kontentkelder (Autodesk Fusion 360 design; units mm, degrees)
Autodesk Fusion 360 part; units mm, degrees
sketch "Sketch1" plane through (0, 0, 0) normal (0, 0, 1) x (1, 0, 0)
  line L0 (0, 0) -> (-148, 0)
  line L1 (-148, 0) -> (-148, 42)
  line L2 (-148, 42) -> (0, 42)
  line L3 (0, 42) -> (0, 0)
  line L4 (-133.4456, 20.7821) -> (-135.5599, 20.7821)
  line L5 (-135.5599, 20.7821) -> (-135.5599, 23.5325)
  line L6 (-135.5599, 23.5325) -> (-136.4022, 23.5325)
  line L7 (-136.4022, 23.5325) -> (-137.9063, 26.7899)
  spline S0 degree 2 poles (-137.9063, 26.7899) (-137.9407, 26.8587) (-138.0524, 27.0563) knots 0 0 0 1 1 1
  spline S1 degree 2 poles (-138.0524, 27.0563) (-138.1126, 27.1595) (-138.3704, 27.6494) knots 0 0 0 1 1 1
  spline S2 degree 2 poles (-138.3704, 27.6494) (-138.8001, 28.4573) (-139.0236, 28.6808) knots 0 0 0 1 1 1
  spline S3 degree 2 poles (-139.0236, 28.6808) (-139.4018, 29.0417) (-140.1323, 29.0503) knots 0 0 0 1 1 1
  line L8 (-140.1323, 29.0503) -> (-140.1323, 23.5325)
  line L9 (-140.1323, 23.5325) -> (-142.6764, 23.5325)
  line L10 (-142.6764, 23.5325) -> (-142.6764, 36.1325)
  line L11 (-142.6764, 36.1325) -> (-140.1323, 36.1325)
  line L12 (-140.1323, 36.1325) -> (-140.1323, 30.7693)
  spline S4 degree 2 poles (-140.1323, 30.7693) (-139.1783, 30.8638) (-138.7228, 31.5514) knots 0 0 0 1 1 1
  spline S5 degree 2 poles (-138.7228, 31.5514) (-138.6111, 31.7405) (-138.0524, 33.1673) knots 0 0 0 1 1 1
  spline S6 degree 2 poles (-138.0524, 33.1673) (-137.3304, 35.0323) (-136.6085, 35.591) knots 0 0 0 1 1 1
  spline S7 degree 2 poles (-136.6085, 35.591) (-135.8091, 36.2098) (-133.9097, 36.2098) knots 0 0 0 1 1 1
  spline S8 degree 2 poles (-133.9097, 36.2098) (-133.8237, 36.2098) (-133.5401, 36.2184) knots 0 0 0 1 1 1
  line L13 (-133.5401, 36.2184) -> (-133.5401, 34.3362)
  line L14 (-133.5401, 34.3362) -> (-133.9011, 34.3447)
  spline S9 degree 2 poles (-133.9011, 34.3447) (-135.1731, 34.3791) (-135.6286, 33.5626) knots 0 0 0 1 1 1
  spline S10 degree 2 poles (-135.6286, 33.5626) (-135.8521, 33.1673) (-136.2905, 31.9382) knots 0 0 0 1 1 1
  spline S11 degree 2 poles (-136.2905, 31.9382) (-136.5655, 31.1647) (-136.8147, 30.8209) knots 0 0 0 1 1 1
  spline S12 degree 2 poles (-136.8147, 30.8209) (-137.1241, 30.3739) (-137.7516, 30.0216) knots 0 0 0 1 1 1
  spline S13 degree 2 poles (-137.7516, 30.0216) (-136.8921, 29.7809) (-136.342, 29.0503) knots 0 0 0 1 1 1
  spline S14 degree 2 poles (-136.342, 29.0503) (-135.7232, 28.2338) (-135.1301, 26.9876) knots 0 0 0 1 1 1
  line L15 (-135.1301, 26.9876) -> (-134.4941, 25.6468)
  line L16 (-134.4941, 25.6468) -> (-133.4456, 25.6468)
  line L17 (-133.4456, 25.6468) -> (-133.4456, 20.7821)
  line L18 (-122.6075, 35.2128) -> (-121.2495, 36.7341)
  line L19 (-121.2495, 36.7341) -> (-120.0548, 35.6855)
  line L20 (-120.0548, 35.6855) -> (-121.4902, 34.0697)
  spline S15 degree 2 poles (-121.4902, 34.0697) (-120.9143, 33.2962) (-120.5963, 32.166) knots 0 0 0 1 1 1
  spline S16 degree 2 poles (-120.5963, 32.166) (-120.2783, 31.0357) (-120.2783, 29.7637) knots 0 0 0 1 1 1
  spline S17 degree 2 poles (-120.2783, 29.7637) (-120.2783, 26.7641) (-121.9371, 25.0409) knots 0 0 0 1 1 1
  spline S18 degree 2 poles (-121.9371, 25.0409) (-123.5959, 23.3176) (-126.3205, 23.3176) knots 0 0 0 1 1 1
  spline S19 degree 2 poles (-126.3205, 23.3176) (-128.684, 23.3176) (-130.1022, 24.392) knots 0 0 0 1 1 1
  line L21 (-130.1022, 24.392) -> (-131.4945, 22.8277)
  line L22 (-131.4945, 22.8277) -> (-132.715, 23.8935)
  line L23 (-132.715, 23.8935) -> (-131.2453, 25.5437)
  spline S20 degree 2 poles (-131.2453, 25.5437) (-132.5001, 27.2196) (-132.5001, 29.9098) knots 0 0 0 1 1 1
  spline S21 degree 2 poles (-132.5001, 29.9098) (-132.5001, 32.8922) (-130.8413, 34.6198) knots 0 0 0 1 1 1
  spline S22 degree 2 poles (-130.8413, 34.6198) (-129.1825, 36.3473) (-126.415, 36.3473) knots 0 0 0 1 1 1
  spline S23 degree 2 poles (-126.415, 36.3473) (-124.1202, 36.3473) (-122.6075, 35.2128) knots 0 0 0 1 1 1
  spline S24 degree 2 poles (-124.1889, 33.4423) (-125.057, 34.1814) (-126.3892, 34.1814) knots 0 0 0 1 1 1
  spline S25 degree 2 poles (-126.3892, 34.1814) (-127.9535, 34.1814) (-128.9161, 33.1028) knots 0 0 0 1 1 1
  spline S26 degree 2 poles (-128.9161, 33.1028) (-129.8787, 32.0241) (-129.8787, 29.8497) knots 0 0 0 1 1 1
  spline S27 degree 2 poles (-129.8787, 29.8497) (-129.8787, 28.4831) (-129.4834, 27.5119) knots 0 0 0 1 1 1
  line L24 (-129.4834, 27.5119) -> (-124.1889, 33.4423)
  line L25 (-123.2521, 32.0929) -> (-128.5379, 26.1539)
  spline S28 degree 2 poles (-128.5379, 26.1539) (-127.6527, 25.3804) (-126.4064, 25.3804) knots 0 0 0 1 1 1
  spline S29 degree 2 poles (-126.4064, 25.3804) (-124.8765, 25.3804) (-123.8924, 26.4891) knots 0 0 0 1 1 1
  spline S30 degree 2 poles (-123.8924, 26.4891) (-122.9083, 27.5978) (-122.9083, 29.7981) knots 0 0 0 1 1 1
  spline S31 degree 2 poles (-122.9083, 29.7981) (-122.9083, 31.1904) (-123.2521, 32.0929) knots 0 0 0 1 1 1
  line L26 (-117.3819, 36.1325) -> (-108.555, 36.1325)
  line L27 (-108.555, 36.1325) -> (-108.555, 23.5325)
  line L28 (-108.555, 23.5325) -> (-111.099, 23.5325)
  line L29 (-111.099, 23.5325) -> (-111.099, 34.001)
  line L30 (-111.099, 34.001) -> (-114.8894, 34.001)
  line L31 (-114.8894, 34.001) -> (-114.8894, 28.6206)
  spline S32 degree 2 poles (-114.8894, 28.6206) (-114.8894, 26.3086) (-115.0441, 25.3932) knots 0 0 0 1 1 1
  spline S33 degree 2 poles (-115.0441, 25.3932) (-115.1988, 24.4779) (-115.7961, 23.9665) knots 0 0 0 1 1 1
  spline S34 degree 2 poles (-115.7961, 23.9665) (-116.3935, 23.4551) (-117.6655, 23.4551) knots 0 0 0 1 1 1
  spline S35 degree 2 poles (-117.6655, 23.4551) (-118.1124, 23.4551) (-119.2899, 23.5411) knots 0 0 0 1 1 1
  line L32 (-119.2899, 23.5411) -> (-119.2899, 25.5093)
  line L33 (-119.2899, 25.5093) -> (-118.7226, 25.5007)
  spline S36 degree 2 poles (-118.7226, 25.5007) (-117.9233, 25.5007) (-117.6483, 25.7156) knots 0 0 0 1 1 1
  spline S37 degree 2 poles (-117.6483, 25.7156) (-117.3733, 25.9304) (-117.3733, 26.7727) knots 0 0 0 1 1 1
  line L34 (-117.3733, 26.7727) -> (-117.3819, 28.9386)
  line L35 (-117.3819, 28.9386) -> (-117.3819, 36.1325)
  line L36 (-103.0973, 23.5325) -> (-103.0973, 34.001)
  line L37 (-103.0973, 34.001) -> (-106.836, 34.001)
  line L38 (-106.836, 34.001) -> (-106.836, 36.1325)
  line L39 (-106.836, 36.1325) -> (-96.8231, 36.1325)
  line L40 (-96.8231, 36.1325) -> (-96.8231, 34.001)
  line L41 (-96.8231, 34.001) -> (-100.5532, 34.001)
  line L42 (-100.5532, 34.001) -> (-100.5532, 23.5325)
  line L43 (-100.5532, 23.5325) -> (-103.0973, 23.5325)
  line L44 (-104.8678, 39.4415) -> (-102.9168, 39.4415)
  line L45 (-102.9168, 39.4415) -> (-101.9885, 38.1608)
  line L46 (-101.9885, 38.1608) -> (-100.9915, 39.4415)
  line L47 (-100.9915, 39.4415) -> (-99.0491, 39.4415)
  line L48 (-99.0491, 39.4415) -> (-100.8282, 36.906)
  line L49 (-100.8282, 36.906) -> (-103.0629, 36.906)
  line L50 (-103.0629, 36.906) -> (-104.8678, 39.4415)
  spline S38 degree 2 poles (-85.8131, 26.4375) (-86.3804, 24.6584) (-87.6008, 23.945) knots 0 0 0 1 1 1
  spline S39 degree 2 poles (-87.6008, 23.945) (-88.6666, 23.3176) (-90.652, 23.3176) knots 0 0 0 1 1 1
  spline S40 degree 2 poles (-90.652, 23.3176) (-92.7061, 23.3176) (-93.9782, 24.1255) knots 0 0 0 1 1 1
  spline S41 degree 2 poles (-93.9782, 24.1255) (-95.508, 25.0881) (-95.508, 27.022) knots 0 0 0 1 1 1
  spline S42 degree 2 poles (-95.508, 27.022) (-95.508, 29.3168) (-92.9984, 30.1763) knots 0 0 0 1 1 1
  spline S43 degree 2 poles (-92.9984, 30.1763) (-95.0611, 31.2764) (-95.0611, 33.0813) knots 0 0 0 1 1 1
  spline S44 degree 2 poles (-95.0611, 33.0813) (-95.0611, 34.7315) (-93.5742, 35.6168) knots 0 0 0 1 1 1
  spline S45 degree 2 poles (-93.5742, 35.6168) (-92.3452, 36.3473) (-90.5832, 36.3473) knots 0 0 0 1 1 1
  spline S46 degree 2 poles (-90.5832, 36.3473) (-86.8359, 36.3473) (-86.0366, 33.2704) knots 0 0 0 1 1 1
  line L51 (-86.0366, 33.2704) -> (-88.5119, 32.6945)
  spline S47 degree 2 poles (-88.5119, 32.6945) (-88.9588, 34.276) (-90.5574, 34.276) knots 0 0 0 1 1 1
  spline S48 degree 2 poles (-90.5574, 34.276) (-91.3739, 34.276) (-91.9068, 33.872) knots 0 0 0 1 1 1
  spline S49 degree 2 poles (-91.9068, 33.872) (-92.4999, 33.4337) (-92.4999, 32.643) knots 0 0 0 1 1 1
  spline S50 degree 2 poles (-92.4999, 32.643) (-92.4999, 31.6632) (-91.7607, 31.1561) knots 0 0 0 1 1 1
  spline S51 degree 2 poles (-91.7607, 31.1561) (-91.1247, 30.7263) (-90.0933, 30.7263) knots 0 0 0 1 1 1
  line L52 (-90.0933, 30.7263) -> (-89.8011, 30.7263)
  line L53 (-89.8011, 30.7263) -> (-89.8011, 28.8269)
  line L54 (-89.8011, 28.8269) -> (-90.3769, 28.8269)
  spline S52 degree 2 poles (-90.3769, 28.8269) (-91.3997, 28.8269) (-92.0443, 28.4831) knots 0 0 0 1 1 1
  spline S53 degree 2 poles (-92.0443, 28.4831) (-92.878, 28.0362) (-92.878, 27.1079) knots 0 0 0 1 1 1
  spline S54 degree 2 poles (-92.878, 27.1079) (-92.878, 26.2312) (-92.1303, 25.7757) knots 0 0 0 1 1 1
  spline S55 degree 2 poles (-92.1303, 25.7757) (-91.5029, 25.3975) (-90.5746, 25.3975) knots 0 0 0 1 1 1
  spline S56 degree 2 poles (-90.5746, 25.3975) (-89.5432, 25.3975) (-89.0018, 25.8015) knots 0 0 0 1 1 1
  spline S57 degree 2 poles (-89.0018, 25.8015) (-88.4603, 26.2055) (-88.1423, 27.2025) knots 0 0 0 1 1 1
  line L55 (-88.1423, 27.2025) -> (-85.8131, 26.4375)
  line L56 (-83.2518, 36.1325) -> (-74.425, 36.1325)
  line L57 (-74.425, 36.1325) -> (-74.425, 23.5325)
  line L58 (-74.425, 23.5325) -> (-76.969, 23.5325)
  line L59 (-76.969, 23.5325) -> (-76.969, 34.001)
  line L60 (-76.969, 34.001) -> (-80.7593, 34.001)
  line L61 (-80.7593, 34.001) -> (-80.7593, 28.6206)
  spline S58 degree 2 poles (-80.7593, 28.6206) (-80.7593, 26.3086) (-80.9141, 25.3932) knots 0 0 0 1 1 1
  spline S59 degree 2 poles (-80.9141, 25.3932) (-81.0688, 24.4779) (-81.6661, 23.9665) knots 0 0 0 1 1 1
  spline S60 degree 2 poles (-81.6661, 23.9665) (-82.2634, 23.4551) (-83.5355, 23.4551) knots 0 0 0 1 1 1
  spline S61 degree 2 poles (-83.5355, 23.4551) (-83.9824, 23.4551) (-85.1599, 23.5411) knots 0 0 0 1 1 1
  line L62 (-85.1599, 23.5411) -> (-85.1599, 25.5093)
  line L63 (-85.1599, 25.5093) -> (-84.5926, 25.5007)
  spline S62 degree 2 poles (-84.5926, 25.5007) (-83.7933, 25.5007) (-83.5183, 25.7156) knots 0 0 0 1 1 1
  spline S63 degree 2 poles (-83.5183, 25.7156) (-83.2432, 25.9304) (-83.2432, 26.7727) knots 0 0 0 1 1 1
  line L64 (-83.2432, 26.7727) -> (-83.2518, 28.9386)
  line L65 (-83.2518, 28.9386) -> (-83.2518, 36.1325)
  line L66 (-68.9673, 23.5325) -> (-68.9673, 34.001)
  line L67 (-68.9673, 34.001) -> (-72.706, 34.001)
  line L68 (-72.706, 34.001) -> (-72.706, 36.1325)
  line L69 (-72.706, 36.1325) -> (-62.693, 36.1325)
  line L70 (-62.693, 36.1325) -> (-62.693, 34.001)
  line L71 (-62.693, 34.001) -> (-66.4232, 34.001)
  line L72 (-66.4232, 34.001) -> (-66.4232, 23.5325)
  line L73 (-66.4232, 23.5325) -> (-68.9673, 23.5325)
  line L74 (-70.7378, 39.4415) -> (-68.7868, 39.4415)
  line L75 (-68.7868, 39.4415) -> (-67.8585, 38.1608)
  line L76 (-67.8585, 38.1608) -> (-66.8615, 39.4415)
  line L77 (-66.8615, 39.4415) -> (-64.9191, 39.4415)
  line L78 (-64.9191, 39.4415) -> (-66.6982, 36.906)
  line L79 (-66.6982, 36.906) -> (-68.9329, 36.906)
  line L80 (-68.9329, 36.906) -> (-70.7378, 39.4415)
  line L81 (-69.8697, 1.1172) -> (-71.984, 1.1172)
  line L82 (-71.984, 1.1172) -> (-71.984, 3.8675)
  line L83 (-71.984, 3.8675) -> (-72.8263, 3.8675)
  line L84 (-72.8263, 3.8675) -> (-74.3304, 7.125)
  spline S64 degree 2 poles (-74.3304, 7.125) (-74.3648, 7.1937) (-74.4765, 7.3914) knots 0 0 0 1 1 1
  spline S65 degree 2 poles (-74.4765, 7.3914) (-74.5367, 7.4945) (-74.7945, 7.9844) knots 0 0 0 1 1 1
  spline S66 degree 2 poles (-74.7945, 7.9844) (-75.2243, 8.7924) (-75.4477, 9.0158) knots 0 0 0 1 1 1
  spline S67 degree 2 poles (-75.4477, 9.0158) (-75.8259, 9.3768) (-76.5565, 9.3854) knots 0 0 0 1 1 1
  line L85 (-76.5565, 9.3854) -> (-76.5565, 3.8675)
  line L86 (-76.5565, 3.8675) -> (-79.1005, 3.8675)
  line L87 (-79.1005, 3.8675) -> (-79.1005, 16.4675)
  line L88 (-79.1005, 16.4675) -> (-76.5565, 16.4675)
  line L89 (-76.5565, 16.4675) -> (-76.5565, 11.1044)
  spline S68 degree 2 poles (-76.5565, 11.1044) (-75.6025, 11.1989) (-75.1469, 11.8865) knots 0 0 0 1 1 1
  spline S69 degree 2 poles (-75.1469, 11.8865) (-75.0352, 12.0756) (-74.4765, 13.5023) knots 0 0 0 1 1 1
  spline S70 degree 2 poles (-74.4765, 13.5023) (-73.7546, 15.3674) (-73.0326, 15.9261) knots 0 0 0 1 1 1
  spline S71 degree 2 poles (-73.0326, 15.9261) (-72.2333, 16.5449) (-70.3338, 16.5449) knots 0 0 0 1 1 1
  spline S72 degree 2 poles (-70.3338, 16.5449) (-70.2479, 16.5449) (-69.9643, 16.5535) knots 0 0 0 1 1 1
  line L90 (-69.9643, 16.5535) -> (-69.9643, 14.6712)
  line L91 (-69.9643, 14.6712) -> (-70.3252, 14.6798)
  spline S73 degree 2 poles (-70.3252, 14.6798) (-71.5973, 14.7142) (-72.0528, 13.8977) knots 0 0 0 1 1 1
  spline S74 degree 2 poles (-72.0528, 13.8977) (-72.2763, 13.5023) (-72.7146, 12.2733) knots 0 0 0 1 1 1
  spline S75 degree 2 poles (-72.7146, 12.2733) (-72.9896, 11.4997) (-73.2389, 11.1559) knots 0 0 0 1 1 1
  spline S76 degree 2 poles (-73.2389, 11.1559) (-73.5483, 10.709) (-74.1757, 10.3566) knots 0 0 0 1 1 1
  spline S77 degree 2 poles (-74.1757, 10.3566) (-73.3162, 10.116) (-72.7662, 9.3854) knots 0 0 0 1 1 1
  spline S78 degree 2 poles (-72.7662, 9.3854) (-72.1473, 8.5689) (-71.5543, 7.3226) knots 0 0 0 1 1 1
  line L92 (-71.5543, 7.3226) -> (-70.9183, 5.9819)
  line L93 (-70.9183, 5.9819) -> (-69.8697, 5.9819)
  line L94 (-69.8697, 5.9819) -> (-69.8697, 1.1172)
  spline S79 degree 2 poles (-59.0317, 6.7726) (-59.5989, 4.9935) (-60.8194, 4.2801) knots 0 0 0 1 1 1
  spline S80 degree 2 poles (-60.8194, 4.2801) (-61.8851, 3.6527) (-63.8705, 3.6527) knots 0 0 0 1 1 1
  spline S81 degree 2 poles (-63.8705, 3.6527) (-65.9247, 3.6527) (-67.1967, 4.4606) knots 0 0 0 1 1 1
  spline S82 degree 2 poles (-67.1967, 4.4606) (-68.7266, 5.4232) (-68.7266, 7.357) knots 0 0 0 1 1 1
  spline S83 degree 2 poles (-68.7266, 7.357) (-68.7266, 9.6518) (-66.2169, 10.5113) knots 0 0 0 1 1 1
  spline S84 degree 2 poles (-66.2169, 10.5113) (-68.2797, 11.6115) (-68.2797, 13.4164) knots 0 0 0 1 1 1
  spline S85 degree 2 poles (-68.2797, 13.4164) (-68.2797, 15.0666) (-66.7928, 15.9518) knots 0 0 0 1 1 1
  spline S86 degree 2 poles (-66.7928, 15.9518) (-65.5637, 16.6824) (-63.8018, 16.6824) knots 0 0 0 1 1 1
  spline S87 degree 2 poles (-63.8018, 16.6824) (-60.0544, 16.6824) (-59.2551, 13.6055) knots 0 0 0 1 1 1
  line L95 (-59.2551, 13.6055) -> (-61.7304, 13.0296)
  spline S88 degree 2 poles (-61.7304, 13.0296) (-62.1774, 14.6111) (-63.776, 14.6111) knots 0 0 0 1 1 1
  spline S89 degree 2 poles (-63.776, 14.6111) (-64.5925, 14.6111) (-65.1254, 14.2071) knots 0 0 0 1 1 1
  spline S90 degree 2 poles (-65.1254, 14.2071) (-65.7184, 13.7688) (-65.7184, 12.978) knots 0 0 0 1 1 1
  spline S91 degree 2 poles (-65.7184, 12.978) (-65.7184, 11.9982) (-64.9793, 11.4911) knots 0 0 0 1 1 1
  spline S92 degree 2 poles (-64.9793, 11.4911) (-64.3433, 11.0614) (-63.3119, 11.0614) knots 0 0 0 1 1 1
  line L96 (-63.3119, 11.0614) -> (-63.0197, 11.0614)
  line L97 (-63.0197, 11.0614) -> (-63.0197, 9.1619)
  line L98 (-63.0197, 9.1619) -> (-63.5955, 9.1619)
  spline S93 degree 2 poles (-63.5955, 9.1619) (-64.6183, 9.1619) (-65.2629, 8.8181) knots 0 0 0 1 1 1
  spline S94 degree 2 poles (-65.2629, 8.8181) (-66.0966, 8.3712) (-66.0966, 7.443) knots 0 0 0 1 1 1
  spline S95 degree 2 poles (-66.0966, 7.443) (-66.0966, 6.5663) (-65.3488, 6.1108) knots 0 0 0 1 1 1
  spline S96 degree 2 poles (-65.3488, 6.1108) (-64.7214, 5.7326) (-63.7932, 5.7326) knots 0 0 0 1 1 1
  spline S97 degree 2 poles (-63.7932, 5.7326) (-62.7618, 5.7326) (-62.2203, 6.1366) knots 0 0 0 1 1 1
  spline S98 degree 2 poles (-62.2203, 6.1366) (-61.6789, 6.5405) (-61.3608, 7.5375) knots 0 0 0 1 1 1
  line L99 (-61.3608, 7.5375) -> (-59.0317, 6.7726)
  line L100 (-57.2353, 10.1589) -> (-57.2353, 16.4675)
  line L101 (-57.2353, 16.4675) -> (-54.6999, 16.4675)
  line L102 (-54.6999, 16.4675) -> (-54.6999, 12.299)
  line L103 (-54.6999, 12.299) -> (-51.8722, 14.6712)
  line L104 (-51.8722, 14.6712) -> (-51.8722, 12.5913)
  line L105 (-51.8722, 12.5913) -> (-54.6999, 10.2277)
  line L106 (-54.6999, 10.2277) -> (-54.6999, 5.9905)
  line L107 (-54.6999, 5.9905) -> (-48.3655, 5.9905)
  line L108 (-48.3655, 5.9905) -> (-48.3655, 3.8675)
  line L109 (-48.3655, 3.8675) -> (-57.2353, 3.8675)
  line L110 (-57.2353, 3.8675) -> (-57.2353, 8.1134)
  line L111 (-57.2353, 8.1134) -> (-58.5675, 7.0046)
  line L112 (-58.5675, 7.0046) -> (-58.5675, 9.0416)
  line L113 (-58.5675, 9.0416) -> (-57.2353, 10.1589)
  line L114 (-46.6207, 16.4675) -> (-41.9795, 16.4675)
  spline S99 degree 2 poles (-41.9795, 16.4675) (-40.3809, 16.4675) (-39.5558, 16.2183) knots 0 0 0 1 1 1
  spline S100 degree 2 poles (-39.5558, 16.2183) (-38.4385, 15.8831) (-37.6478, 15.0365) knots 0 0 0 1 1 1
  spline S101 degree 2 poles (-37.6478, 15.0365) (-36.857, 14.1899) (-36.4574, 12.9866) knots 0 0 0 1 1 1
  spline S102 degree 2 poles (-36.4574, 12.9866) (-36.0577, 11.7834) (-36.0577, 10.0128) knots 0 0 0 1 1 1
  spline S103 degree 2 poles (-36.0577, 10.0128) (-36.0577, 8.4572) (-36.5003, 7.2066) knots 0 0 0 1 1 1
  spline S104 degree 2 poles (-36.5003, 7.2066) (-36.943, 5.9561) (-37.8025, 5.1224) knots 0 0 0 1 1 1
  spline S105 degree 2 poles (-37.8025, 5.1224) (-38.4643, 4.495) (-39.5816, 4.134) knots 0 0 0 1 1 1
  spline S106 degree 2 poles (-39.5816, 4.134) (-40.4239, 3.8675) (-41.842, 3.8675) knots 0 0 0 1 1 1
  line L115 (-41.842, 3.8675) -> (-46.6207, 3.8675)
  line L116 (-46.6207, 3.8675) -> (-46.6207, 9.3682)
  line L117 (-46.6207, 9.3682) -> (-47.9272, 9.3682)
  line L118 (-47.9272, 9.3682) -> (-47.9272, 10.9668)
  line L119 (-47.9272, 10.9668) -> (-46.6207, 10.9668)
  line L120 (-46.6207, 10.9668) -> (-46.6207, 16.4675)
  line L121 (-44.0853, 14.336) -> (-44.0853, 10.9668)
  line L122 (-44.0853, 10.9668) -> (-41.3865, 10.9668)
  line L123 (-41.3865, 10.9668) -> (-41.3865, 9.3682)
  line L124 (-41.3865, 9.3682) -> (-44.0853, 9.3682)
  line L125 (-44.0853, 9.3682) -> (-44.0853, 5.9905)
  line L126 (-44.0853, 5.9905) -> (-42.1772, 5.9905)
  spline S107 degree 2 poles (-42.1772, 5.9905) (-40.9138, 5.9905) (-40.3551, 6.1967) knots 0 0 0 1 1 1
  spline S108 degree 2 poles (-40.3551, 6.1967) (-39.616, 6.4546) (-39.2292, 7.1422) knots 0 0 0 1 1 1
  spline S109 degree 2 poles (-39.2292, 7.1422) (-38.6877, 8.1134) (-38.6877, 10.1074) knots 0 0 0 1 1 1
  spline S110 degree 2 poles (-38.6877, 10.1074) (-38.6877, 11.5255) (-38.9155, 12.2947) knots 0 0 0 1 1 1
  spline S111 degree 2 poles (-38.9155, 12.2947) (-39.1433, 13.064) (-39.5859, 13.5367) knots 0 0 0 1 1 1
  spline S112 degree 2 poles (-39.5859, 13.5367) (-40.0285, 14.0094) (-40.7419, 14.1985) knots 0 0 0 1 1 1
  spline S113 degree 2 poles (-40.7419, 14.1985) (-41.292, 14.336) (-42.9336, 14.336) knots 0 0 0 1 1 1
  line L127 (-42.9336, 14.336) -> (-44.0853, 14.336)
  spline S114 degree 2 poles (-24.5407, 6.7726) (-25.1079, 4.9935) (-26.3284, 4.2801) knots 0 0 0 1 1 1
  spline S115 degree 2 poles (-26.3284, 4.2801) (-27.3941, 3.6527) (-29.3795, 3.6527) knots 0 0 0 1 1 1
  spline S116 degree 2 poles (-29.3795, 3.6527) (-31.4337, 3.6527) (-32.7057, 4.4606) knots 0 0 0 1 1 1
  spline S117 degree 2 poles (-32.7057, 4.4606) (-34.2356, 5.4232) (-34.2356, 7.357) knots 0 0 0 1 1 1
  spline S118 degree 2 poles (-34.2356, 7.357) (-34.2356, 9.6518) (-31.7259, 10.5113) knots 0 0 0 1 1 1
  spline S119 degree 2 poles (-31.7259, 10.5113) (-33.7887, 11.6115) (-33.7887, 13.4164) knots 0 0 0 1 1 1
  spline S120 degree 2 poles (-33.7887, 13.4164) (-33.7887, 15.0666) (-32.3018, 15.9518) knots 0 0 0 1 1 1
  spline S121 degree 2 poles (-32.3018, 15.9518) (-31.0727, 16.6824) (-29.3108, 16.6824) knots 0 0 0 1 1 1
  spline S122 degree 2 poles (-29.3108, 16.6824) (-25.5634, 16.6824) (-24.7641, 13.6055) knots 0 0 0 1 1 1
  line L128 (-24.7641, 13.6055) -> (-27.2394, 13.0296)
  spline S123 degree 2 poles (-27.2394, 13.0296) (-27.6864, 14.6111) (-29.285, 14.6111) knots 0 0 0 1 1 1
  spline S124 degree 2 poles (-29.285, 14.6111) (-30.1015, 14.6111) (-30.6344, 14.2071) knots 0 0 0 1 1 1
  spline S125 degree 2 poles (-30.6344, 14.2071) (-31.2274, 13.7688) (-31.2274, 12.978) knots 0 0 0 1 1 1
  spline S126 degree 2 poles (-31.2274, 12.978) (-31.2274, 11.9982) (-30.4883, 11.4911) knots 0 0 0 1 1 1
  spline S127 degree 2 poles (-30.4883, 11.4911) (-29.8523, 11.0614) (-28.8209, 11.0614) knots 0 0 0 1 1 1
  line L129 (-28.8209, 11.0614) -> (-28.5286, 11.0614)
  line L130 (-28.5286, 11.0614) -> (-28.5286, 9.1619)
  line L131 (-28.5286, 9.1619) -> (-29.1045, 9.1619)
  spline S128 degree 2 poles (-29.1045, 9.1619) (-30.1273, 9.1619) (-30.7719, 8.8181) knots 0 0 0 1 1 1
  spline S129 degree 2 poles (-30.7719, 8.8181) (-31.6056, 8.3712) (-31.6056, 7.443) knots 0 0 0 1 1 1
  spline S130 degree 2 poles (-31.6056, 7.443) (-31.6056, 6.5663) (-30.8578, 6.1108) knots 0 0 0 1 1 1
  spline S131 degree 2 poles (-30.8578, 6.1108) (-30.2304, 5.7326) (-29.3022, 5.7326) knots 0 0 0 1 1 1
  spline S132 degree 2 poles (-29.3022, 5.7326) (-28.2708, 5.7326) (-27.7293, 6.1366) knots 0 0 0 1 1 1
  spline S133 degree 2 poles (-27.7293, 6.1366) (-27.1879, 6.5405) (-26.8698, 7.5375) knots 0 0 0 1 1 1
  line L132 (-26.8698, 7.5375) -> (-24.5407, 6.7726)
  line L133 (-15.5741, 10.6467) -> (-18.8283, 10.6467)
  line L134 (-18.8283, 10.6467) -> (-18.8283, 9.8721)
  spline S134 degree 2 poles (-18.8283, 9.8721) (-18.8283, 5.7476) (-21.9192, 2.3172) knots 0 0 0 1 1 1
  line L135 (-21.9192, 2.3172) -> (-23.4212, 3.7107)
  spline S135 degree 2 poles (-23.4212, 3.7107) (-20.89, 6.2032) (-20.89, 10.8154) knots 0 0 0 1 1 1
  line L136 (-20.89, 10.8154) -> (-20.89, 17.1551)
  line L137 (-20.89, 17.1551) -> (-9.2559, 17.1551)
  line L138 (-9.2559, 17.1551) -> (-9.2559, 10.0698)
  line L139 (-9.2559, 10.0698) -> (-11.3175, 10.0698)
  line L140 (-11.3175, 10.0698) -> (-11.3175, 10.6467)
  line L141 (-11.3175, 10.6467) -> (-13.7724, 10.6467)
  line L142 (-13.7724, 10.6467) -> (-13.65, 10.2696)
  spline S136 degree 2 poles (-13.65, 10.2696) (-12.9817, 6.5867) (-7.5025, 4.683) knots 0 0 0 1 1 1
  line L143 (-7.5025, 4.683) -> (-8.1192, 2.7212)
  spline S137 degree 2 poles (-8.1192, 2.7212) (-14.8425, 4.9977) (-15.5333, 10.3803) knots 0 0 0 1 1 1
  line L144 (-15.5333, 10.3803) -> (-15.5741, 10.6467)
  line L145 (-11.3175, 12.5709) -> (-11.3175, 15.231)
  line L146 (-11.3175, 15.231) -> (-18.8283, 15.231)
  line L147 (-18.8283, 15.231) -> (-18.8283, 12.5709)
  line L148 (-18.8283, 12.5709) -> (-11.3175, 12.5709)
  dimension "d1" = 42
  dimension "d2" = 148
  constraint horizontal L0
  constraint vertical L1
  constraint horizontal L2
  constraint vertical L3
  constraint coincident L0.start L3.end
  measures "d1" distance of L0.start L2.end
  measures "d2" distance of L1.end L2.end
extrude "Extrude1" add sketch "Sketch1" against normal blind 10 makes body 1 at (-16.3247, 12.5709, -3.3333) makes body 2 at (-42.8018, 12.0899, 0) makes body 3 at (-127.7186, 29.4887, -3.3333) makes body 4 at (-30.8238, 31.6005, 0) makes body 5 at (-125.0141, 30.1132, -3.3333)
sketch "Sketch2" plane through (0, 0, -10) normal (0, 0, -1) x (1, 0, 0)
  spline S0 degree 2 poles (-126.415, -36.3473) (-129.1825, -36.3473) (-130.8413, -34.6198) knots -1 -1 -1 0 0 0
  spline S1 degree 2 poles (-130.8413, -34.6198) (-132.5001, -32.8922) (-132.5001, -29.9098) knots -1 -1 -1 0 0 0
  spline S2 degree 2 poles (-132.5001, -29.9098) (-132.5001, -27.2196) (-131.2453, -25.5437) knots -1 -1 -1 0 0 0
  line L0 (-131.2453, -25.5437) -> (-132.715, -23.8935)
  line L1 (-132.715, -23.8935) -> (-131.4945, -22.8277)
  line L2 (-131.4945, -22.8277) -> (-130.1022, -24.392)
  spline S3 degree 2 poles (-130.1022, -24.392) (-128.684, -23.3176) (-126.3205, -23.3176) knots -1 -1 -1 0 0 0
  spline S4 degree 2 poles (-126.3205, -23.3176) (-123.5959, -23.3176) (-121.9371, -25.0409) knots -1 -1 -1 0 0 0
  spline S5 degree 2 poles (-121.9371, -25.0409) (-120.2783, -26.7641) (-120.2783, -29.7637) knots -1 -1 -1 0 0 0
  spline S6 degree 2 poles (-120.2783, -29.7637) (-120.2783, -31.0357) (-120.5963, -32.166) knots -1 -1 -1 0 0 0
  spline S7 degree 2 poles (-120.5963, -32.166) (-120.9143, -33.2962) (-121.4902, -34.0697) knots -1 -1 -1 0 0 0
  line L3 (-121.4902, -34.0697) -> (-120.0548, -35.6855)
  line L4 (-120.0548, -35.6855) -> (-121.2495, -36.7341)
  line L5 (-121.2495, -36.7341) -> (-122.6075, -35.2128)
  spline S8 degree 2 poles (-122.6075, -35.2128) (-124.1202, -36.3473) (-126.415, -36.3473) knots -1 -1 -1 0 0 0
  line L6 (-117.3819, -28.9386) -> (-117.3733, -26.7727)
  spline S9 degree 2 poles (-117.3733, -26.7727) (-117.3733, -25.9304) (-117.6483, -25.7156) knots -1 -1 -1 0 0 0
  spline S10 degree 2 poles (-117.6483, -25.7156) (-117.9233, -25.5007) (-118.7226, -25.5007) knots -1 -1 -1 0 0 0
  line L7 (-118.7226, -25.5007) -> (-119.2899, -25.5093)
  line L8 (-119.2899, -25.5093) -> (-119.2899, -23.5411)
  spline S11 degree 2 poles (-119.2899, -23.5411) (-118.1124, -23.4551) (-117.6655, -23.4551) knots -1 -1 -1 0 0 0
  spline S12 degree 2 poles (-117.6655, -23.4551) (-116.3935, -23.4551) (-115.7961, -23.9665) knots -1 -1 -1 0 0 0
  spline S13 degree 2 poles (-115.7961, -23.9665) (-115.1988, -24.4779) (-115.0441, -25.3932) knots -1 -1 -1 0 0 0
  spline S14 degree 2 poles (-115.0441, -25.3932) (-114.8894, -26.3086) (-114.8894, -28.6206) knots -1 -1 -1 0 0 0
  line L9 (-114.8894, -28.6206) -> (-114.8894, -34.001)
  line L10 (-114.8894, -34.001) -> (-111.099, -34.001)
  line L11 (-111.099, -34.001) -> (-111.099, -23.5325)
  line L12 (-111.099, -23.5325) -> (-108.555, -23.5325)
  line L13 (-108.555, -23.5325) -> (-108.555, -36.1325)
  line L14 (-108.555, -36.1325) -> (-117.3819, -36.1325)
  line L15 (-117.3819, -36.1325) -> (-117.3819, -28.9386)
  line L16 (-103.0629, -36.906) -> (-100.8282, -36.906)
  line L17 (-100.8282, -36.906) -> (-99.0491, -39.4415)
  line L18 (-99.0491, -39.4415) -> (-100.9915, -39.4415)
  line L19 (-100.9915, -39.4415) -> (-101.9885, -38.1608)
  line L20 (-101.9885, -38.1608) -> (-102.9168, -39.4415)
  line L21 (-102.9168, -39.4415) -> (-104.8678, -39.4415)
  line L22 (-104.8678, -39.4415) -> (-103.0629, -36.906)
  spline S15 degree 2 poles (-88.1423, -27.2025) (-88.4603, -26.2055) (-89.0018, -25.8015) knots -1 -1 -1 0 0 0
  spline S16 degree 2 poles (-89.0018, -25.8015) (-89.5432, -25.3975) (-90.5746, -25.3975) knots -1 -1 -1 0 0 0
  spline S17 degree 2 poles (-90.5746, -25.3975) (-91.5029, -25.3975) (-92.1303, -25.7757) knots -1 -1 -1 0 0 0
  spline S18 degree 2 poles (-92.1303, -25.7757) (-92.878, -26.2312) (-92.878, -27.1079) knots -1 -1 -1 0 0 0
  spline S19 degree 2 poles (-92.878, -27.1079) (-92.878, -28.0362) (-92.0443, -28.4831) knots -1 -1 -1 0 0 0
  spline S20 degree 2 poles (-92.0443, -28.4831) (-91.3997, -28.8269) (-90.3769, -28.8269) knots -1 -1 -1 0 0 0
  line L23 (-90.3769, -28.8269) -> (-89.8011, -28.8269)
  line L24 (-89.8011, -28.8269) -> (-89.8011, -30.7263)
  line L25 (-89.8011, -30.7263) -> (-90.0933, -30.7263)
  spline S21 degree 2 poles (-90.0933, -30.7263) (-91.1247, -30.7263) (-91.7607, -31.1561) knots -1 -1 -1 0 0 0
  spline S22 degree 2 poles (-91.7607, -31.1561) (-92.4999, -31.6632) (-92.4999, -32.643) knots -1 -1 -1 0 0 0
  spline S23 degree 2 poles (-92.4999, -32.643) (-92.4999, -33.4337) (-91.9068, -33.872) knots -1 -1 -1 0 0 0
  spline S24 degree 2 poles (-91.9068, -33.872) (-91.3739, -34.276) (-90.5574, -34.276) knots -1 -1 -1 0 0 0
  spline S25 degree 2 poles (-90.5574, -34.276) (-88.9588, -34.276) (-88.5119, -32.6945) knots -1 -1 -1 0 0 0
  line L26 (-88.5119, -32.6945) -> (-86.0366, -33.2704)
  spline S26 degree 2 poles (-86.0366, -33.2704) (-86.8359, -36.3473) (-90.5832, -36.3473) knots -1 -1 -1 0 0 0
  spline S27 degree 2 poles (-90.5832, -36.3473) (-92.3452, -36.3473) (-93.5742, -35.6168) knots -1 -1 -1 0 0 0
  spline S28 degree 2 poles (-93.5742, -35.6168) (-95.0611, -34.7315) (-95.0611, -33.0813) knots -1 -1 -1 0 0 0
  spline S29 degree 2 poles (-95.0611, -33.0813) (-95.0611, -31.2764) (-92.9984, -30.1763) knots -1 -1 -1 0 0 0
  spline S30 degree 2 poles (-92.9984, -30.1763) (-95.508, -29.3168) (-95.508, -27.022) knots -1 -1 -1 0 0 0
  spline S31 degree 2 poles (-95.508, -27.022) (-95.508, -25.0881) (-93.9782, -24.1255) knots -1 -1 -1 0 0 0
  spline S32 degree 2 poles (-93.9782, -24.1255) (-92.7061, -23.3176) (-90.652, -23.3176) knots -1 -1 -1 0 0 0
  spline S33 degree 2 poles (-90.652, -23.3176) (-88.6666, -23.3176) (-87.6008, -23.945) knots -1 -1 -1 0 0 0
  spline S34 degree 2 poles (-87.6008, -23.945) (-86.3804, -24.6584) (-85.8131, -26.4375) knots -1 -1 -1 0 0 0
  line L27 (-85.8131, -26.4375) -> (-88.1423, -27.2025)
  line L28 (-100.5532, -23.5325) -> (-100.5532, -34.001)
  line L29 (-100.5532, -34.001) -> (-96.8231, -34.001)
  line L30 (-96.8231, -34.001) -> (-96.8231, -36.1325)
  line L31 (-96.8231, -36.1325) -> (-106.836, -36.1325)
  line L32 (-106.836, -36.1325) -> (-106.836, -34.001)
  line L33 (-106.836, -34.001) -> (-103.0973, -34.001)
  line L34 (-103.0973, -34.001) -> (-103.0973, -23.5325)
  line L35 (-103.0973, -23.5325) -> (-100.5532, -23.5325)
  line L36 (-68.9329, -36.906) -> (-66.6982, -36.906)
  line L37 (-66.6982, -36.906) -> (-64.9191, -39.4415)
  line L38 (-64.9191, -39.4415) -> (-66.8615, -39.4415)
  line L39 (-66.8615, -39.4415) -> (-67.8585, -38.1608)
  line L40 (-67.8585, -38.1608) -> (-68.7868, -39.4415)
  line L41 (-68.7868, -39.4415) -> (-70.7378, -39.4415)
  line L42 (-70.7378, -39.4415) -> (-68.9329, -36.906)
  line L43 (-69.8697, -5.9819) -> (-70.9183, -5.9819)
  line L44 (-70.9183, -5.9819) -> (-71.5543, -7.3226)
  spline S35 degree 2 poles (-71.5543, -7.3226) (-72.1473, -8.5689) (-72.7662, -9.3854) knots -1 -1 -1 0 0 0
  spline S36 degree 2 poles (-72.7662, -9.3854) (-73.3162, -10.116) (-74.1757, -10.3566) knots -1 -1 -1 0 0 0
  spline S37 degree 2 poles (-74.1757, -10.3566) (-73.5483, -10.709) (-73.2389, -11.1559) knots -1 -1 -1 0 0 0
  spline S38 degree 2 poles (-73.2389, -11.1559) (-72.9896, -11.4997) (-72.7146, -12.2733) knots -1 -1 -1 0 0 0
  spline S39 degree 2 poles (-72.7146, -12.2733) (-72.2763, -13.5023) (-72.0528, -13.8977) knots -1 -1 -1 0 0 0
  spline S40 degree 2 poles (-72.0528, -13.8977) (-71.5973, -14.7142) (-70.3252, -14.6798) knots -1 -1 -1 0 0 0
  line L45 (-70.3252, -14.6798) -> (-69.9643, -14.6712)
  line L46 (-69.9643, -14.6712) -> (-69.9643, -16.5535)
  spline S41 degree 2 poles (-69.9643, -16.5535) (-70.2479, -16.5449) (-70.3338, -16.5449) knots -1 -1 -1 0 0 0
  spline S42 degree 2 poles (-70.3338, -16.5449) (-72.2333, -16.5449) (-73.0326, -15.9261) knots -1 -1 -1 0 0 0
  spline S43 degree 2 poles (-73.0326, -15.9261) (-73.7546, -15.3674) (-74.4765, -13.5023) knots -1 -1 -1 0 0 0
  spline S44 degree 2 poles (-74.4765, -13.5023) (-75.0352, -12.0756) (-75.1469, -11.8865) knots -1 -1 -1 0 0 0
  spline S45 degree 2 poles (-75.1469, -11.8865) (-75.6025, -11.1989) (-76.5565, -11.1044) knots -1 -1 -1 0 0 0
  line L47 (-76.5565, -11.1044) -> (-76.5565, -16.4675)
  line L48 (-76.5565, -16.4675) -> (-79.1005, -16.4675)
  line L49 (-79.1005, -16.4675) -> (-79.1005, -3.8675)
  line L50 (-79.1005, -3.8675) -> (-76.5565, -3.8675)
  line L51 (-76.5565, -3.8675) -> (-76.5565, -9.3854)
  spline S46 degree 2 poles (-76.5565, -9.3854) (-75.8259, -9.3768) (-75.4477, -9.0158) knots -1 -1 -1 0 0 0
  spline S47 degree 2 poles (-75.4477, -9.0158) (-75.2243, -8.7924) (-74.7945, -7.9844) knots -1 -1 -1 0 0 0
  spline S48 degree 2 poles (-74.7945, -7.9844) (-74.5367, -7.4945) (-74.4765, -7.3914) knots -1 -1 -1 0 0 0
  spline S49 degree 2 poles (-74.4765, -7.3914) (-74.3648, -7.1937) (-74.3304, -7.125) knots -1 -1 -1 0 0 0
  line L52 (-74.3304, -7.125) -> (-72.8263, -3.8675)
  line L53 (-72.8263, -3.8675) -> (-71.984, -3.8675)
  line L54 (-71.984, -3.8675) -> (-71.984, -1.1172)
  line L55 (-71.984, -1.1172) -> (-69.8697, -1.1172)
  line L56 (-69.8697, -1.1172) -> (-69.8697, -5.9819)
  line L57 (-83.2518, -28.9386) -> (-83.2432, -26.7727)
  spline S50 degree 2 poles (-83.2432, -26.7727) (-83.2432, -25.9304) (-83.5183, -25.7156) knots -1 -1 -1 0 0 0
  spline S51 degree 2 poles (-83.5183, -25.7156) (-83.7933, -25.5007) (-84.5926, -25.5007) knots -1 -1 -1 0 0 0
  line L58 (-84.5926, -25.5007) -> (-85.1599, -25.5093)
  line L59 (-85.1599, -25.5093) -> (-85.1599, -23.5411)
  spline S52 degree 2 poles (-85.1599, -23.5411) (-83.9824, -23.4551) (-83.5355, -23.4551) knots -1 -1 -1 0 0 0
  spline S53 degree 2 poles (-83.5355, -23.4551) (-82.2634, -23.4551) (-81.6661, -23.9665) knots -1 -1 -1 0 0 0
  spline S54 degree 2 poles (-81.6661, -23.9665) (-81.0688, -24.4779) (-80.9141, -25.3932) knots -1 -1 -1 0 0 0
  spline S55 degree 2 poles (-80.9141, -25.3932) (-80.7593, -26.3086) (-80.7593, -28.6206) knots -1 -1 -1 0 0 0
  line L60 (-80.7593, -28.6206) -> (-80.7593, -34.001)
  line L61 (-80.7593, -34.001) -> (-76.969, -34.001)
  line L62 (-76.969, -34.001) -> (-76.969, -23.5325)
  line L63 (-76.969, -23.5325) -> (-74.425, -23.5325)
  line L64 (-74.425, -23.5325) -> (-74.425, -36.1325)
  line L65 (-74.425, -36.1325) -> (-83.2518, -36.1325)
  line L66 (-83.2518, -36.1325) -> (-83.2518, -28.9386)
  line L67 (-66.4232, -23.5325) -> (-66.4232, -34.001)
  line L68 (-66.4232, -34.001) -> (-62.693, -34.001)
  line L69 (-62.693, -34.001) -> (-62.693, -36.1325)
  line L70 (-62.693, -36.1325) -> (-72.706, -36.1325)
  line L71 (-72.706, -36.1325) -> (-72.706, -34.001)
  line L72 (-72.706, -34.001) -> (-68.9673, -34.001)
  line L73 (-68.9673, -34.001) -> (-68.9673, -23.5325)
  line L74 (-68.9673, -23.5325) -> (-66.4232, -23.5325)
  spline S56 degree 2 poles (-61.3608, -7.5375) (-61.6789, -6.5405) (-62.2203, -6.1366) knots -1 -1 -1 0 0 0
  spline S57 degree 2 poles (-62.2203, -6.1366) (-62.7618, -5.7326) (-63.7932, -5.7326) knots -1 -1 -1 0 0 0
  spline S58 degree 2 poles (-63.7932, -5.7326) (-64.7214, -5.7326) (-65.3488, -6.1108) knots -1 -1 -1 0 0 0
  spline S59 degree 2 poles (-65.3488, -6.1108) (-66.0966, -6.5663) (-66.0966, -7.443) knots -1 -1 -1 0 0 0
  spline S60 degree 2 poles (-66.0966, -7.443) (-66.0966, -8.3712) (-65.2629, -8.8181) knots -1 -1 -1 0 0 0
  spline S61 degree 2 poles (-65.2629, -8.8181) (-64.6183, -9.1619) (-63.5955, -9.1619) knots -1 -1 -1 0 0 0
  line L75 (-63.5955, -9.1619) -> (-63.0197, -9.1619)
  line L76 (-63.0197, -9.1619) -> (-63.0197, -11.0614)
  line L77 (-63.0197, -11.0614) -> (-63.3119, -11.0614)
  spline S62 degree 2 poles (-63.3119, -11.0614) (-64.3433, -11.0614) (-64.9793, -11.4911) knots -1 -1 -1 0 0 0
  spline S63 degree 2 poles (-64.9793, -11.4911) (-65.7184, -11.9982) (-65.7184, -12.978) knots -1 -1 -1 0 0 0
  spline S64 degree 2 poles (-65.7184, -12.978) (-65.7184, -13.7688) (-65.1254, -14.2071) knots -1 -1 -1 0 0 0
  spline S65 degree 2 poles (-65.1254, -14.2071) (-64.5925, -14.6111) (-63.776, -14.6111) knots -1 -1 -1 0 0 0
  spline S66 degree 2 poles (-63.776, -14.6111) (-62.1774, -14.6111) (-61.7304, -13.0296) knots -1 -1 -1 0 0 0
  line L78 (-61.7304, -13.0296) -> (-59.2551, -13.6055)
  spline S67 degree 2 poles (-59.2551, -13.6055) (-60.0544, -16.6824) (-63.8018, -16.6824) knots -1 -1 -1 0 0 0
  spline S68 degree 2 poles (-63.8018, -16.6824) (-65.5637, -16.6824) (-66.7928, -15.9518) knots -1 -1 -1 0 0 0
  spline S69 degree 2 poles (-66.7928, -15.9518) (-68.2797, -15.0666) (-68.2797, -13.4164) knots -1 -1 -1 0 0 0
  spline S70 degree 2 poles (-68.2797, -13.4164) (-68.2797, -11.6115) (-66.2169, -10.5113) knots -1 -1 -1 0 0 0
  spline S71 degree 2 poles (-66.2169, -10.5113) (-68.7266, -9.6518) (-68.7266, -7.357) knots -1 -1 -1 0 0 0
  spline S72 degree 2 poles (-68.7266, -7.357) (-68.7266, -5.4232) (-67.1967, -4.4606) knots -1 -1 -1 0 0 0
  spline S73 degree 2 poles (-67.1967, -4.4606) (-65.9247, -3.6527) (-63.8705, -3.6527) knots -1 -1 -1 0 0 0
  spline S74 degree 2 poles (-63.8705, -3.6527) (-61.8851, -3.6527) (-60.8194, -4.2801) knots -1 -1 -1 0 0 0
  spline S75 degree 2 poles (-60.8194, -4.2801) (-59.5989, -4.9935) (-59.0317, -6.7726) knots -1 -1 -1 0 0 0
  line L79 (-59.0317, -6.7726) -> (-61.3608, -7.5375)
  line L80 (-46.6207, -10.9668) -> (-47.9272, -10.9668)
  line L81 (-47.9272, -10.9668) -> (-47.9272, -9.3682)
  line L82 (-47.9272, -9.3682) -> (-46.6207, -9.3682)
  line L83 (-46.6207, -9.3682) -> (-46.6207, -3.8675)
  line L84 (-46.6207, -3.8675) -> (-41.842, -3.8675)
  spline S76 degree 2 poles (-41.842, -3.8675) (-40.4239, -3.8675) (-39.5816, -4.134) knots -1 -1 -1 0 0 0
  spline S77 degree 2 poles (-39.5816, -4.134) (-38.4643, -4.495) (-37.8025, -5.1224) knots -1 -1 -1 0 0 0
  spline S78 degree 2 poles (-37.8025, -5.1224) (-36.943, -5.9561) (-36.5003, -7.2066) knots -1 -1 -1 0 0 0
  spline S79 degree 2 poles (-36.5003, -7.2066) (-36.0577, -8.4572) (-36.0577, -10.0128) knots -1 -1 -1 0 0 0
  spline S80 degree 2 poles (-36.0577, -10.0128) (-36.0577, -11.7834) (-36.4574, -12.9866) knots -1 -1 -1 0 0 0
  spline S81 degree 2 poles (-36.4574, -12.9866) (-36.857, -14.1899) (-37.6478, -15.0365) knots -1 -1 -1 0 0 0
  spline S82 degree 2 poles (-37.6478, -15.0365) (-38.4385, -15.8831) (-39.5558, -16.2183) knots -1 -1 -1 0 0 0
  spline S83 degree 2 poles (-39.5558, -16.2183) (-40.3809, -16.4675) (-41.9795, -16.4675) knots -1 -1 -1 0 0 0
  line L85 (-41.9795, -16.4675) -> (-46.6207, -16.4675)
  line L86 (-46.6207, -16.4675) -> (-46.6207, -10.9668)
  spline S84 degree 2 poles (-26.8698, -7.5375) (-27.1879, -6.5405) (-27.7293, -6.1366) knots -1 -1 -1 0 0 0
  spline S85 degree 2 poles (-27.7293, -6.1366) (-28.2708, -5.7326) (-29.3022, -5.7326) knots -1 -1 -1 0 0 0
  spline S86 degree 2 poles (-29.3022, -5.7326) (-30.2304, -5.7326) (-30.8578, -6.1108) knots -1 -1 -1 0 0 0
  spline S87 degree 2 poles (-30.8578, -6.1108) (-31.6056, -6.5663) (-31.6056, -7.443) knots -1 -1 -1 0 0 0
  spline S88 degree 2 poles (-31.6056, -7.443) (-31.6056, -8.3712) (-30.7719, -8.8181) knots -1 -1 -1 0 0 0
  spline S89 degree 2 poles (-30.7719, -8.8181) (-30.1273, -9.1619) (-29.1045, -9.1619) knots -1 -1 -1 0 0 0
  line L87 (-29.1045, -9.1619) -> (-28.5286, -9.1619)
  line L88 (-28.5286, -9.1619) -> (-28.5286, -11.0614)
  line L89 (-28.5286, -11.0614) -> (-28.8209, -11.0614)
  spline S90 degree 2 poles (-28.8209, -11.0614) (-29.8523, -11.0614) (-30.4883, -11.4911) knots -1 -1 -1 0 0 0
  spline S91 degree 2 poles (-30.4883, -11.4911) (-31.2274, -11.9982) (-31.2274, -12.978) knots -1 -1 -1 0 0 0
  spline S92 degree 2 poles (-31.2274, -12.978) (-31.2274, -13.7688) (-30.6344, -14.2071) knots -1 -1 -1 0 0 0
  spline S93 degree 2 poles (-30.6344, -14.2071) (-30.1015, -14.6111) (-29.285, -14.6111) knots -1 -1 -1 0 0 0
  spline S94 degree 2 poles (-29.285, -14.6111) (-27.6864, -14.6111) (-27.2394, -13.0296) knots -1 -1 -1 0 0 0
  line L90 (-27.2394, -13.0296) -> (-24.7641, -13.6055)
  spline S95 degree 2 poles (-24.7641, -13.6055) (-25.5634, -16.6824) (-29.3108, -16.6824) knots -1 -1 -1 0 0 0
  spline S96 degree 2 poles (-29.3108, -16.6824) (-31.0727, -16.6824) (-32.3018, -15.9518) knots -1 -1 -1 0 0 0
  spline S97 degree 2 poles (-32.3018, -15.9518) (-33.7887, -15.0666) (-33.7887, -13.4164) knots -1 -1 -1 0 0 0
  spline S98 degree 2 poles (-33.7887, -13.4164) (-33.7887, -11.6115) (-31.7259, -10.5113) knots -1 -1 -1 0 0 0
  spline S99 degree 2 poles (-31.7259, -10.5113) (-34.2356, -9.6518) (-34.2356, -7.357) knots -1 -1 -1 0 0 0
  spline S100 degree 2 poles (-34.2356, -7.357) (-34.2356, -5.4232) (-32.7057, -4.4606) knots -1 -1 -1 0 0 0
  spline S101 degree 2 poles (-32.7057, -4.4606) (-31.4337, -3.6527) (-29.3795, -3.6527) knots -1 -1 -1 0 0 0
  spline S102 degree 2 poles (-29.3795, -3.6527) (-27.3941, -3.6527) (-26.3284, -4.2801) knots -1 -1 -1 0 0 0
  spline S103 degree 2 poles (-26.3284, -4.2801) (-25.1079, -4.9935) (-24.5407, -6.7726) knots -1 -1 -1 0 0 0
  line L91 (-24.5407, -6.7726) -> (-26.8698, -7.5375)
  line L92 (-58.5675, -9.0416) -> (-58.5675, -7.0046)
  line L93 (-58.5675, -7.0046) -> (-57.2353, -8.1134)
  line L94 (-57.2353, -8.1134) -> (-57.2353, -3.8675)
  line L95 (-57.2353, -3.8675) -> (-48.3655, -3.8675)
  line L96 (-48.3655, -3.8675) -> (-48.3655, -5.9905)
  line L97 (-48.3655, -5.9905) -> (-54.6999, -5.9905)
  line L98 (-54.6999, -5.9905) -> (-54.6999, -10.2277)
  line L99 (-54.6999, -10.2277) -> (-51.8722, -12.5913)
  line L100 (-51.8722, -12.5913) -> (-51.8722, -14.6712)
  line L101 (-51.8722, -14.6712) -> (-54.6999, -12.299)
  line L102 (-54.6999, -12.299) -> (-54.6999, -16.4675)
  line L103 (-54.6999, -16.4675) -> (-57.2353, -16.4675)
  line L104 (-57.2353, -16.4675) -> (-57.2353, -10.1589)
  line L105 (-57.2353, -10.1589) -> (-58.5675, -9.0416)
  spline S104 degree 2 poles (-15.5333, -10.3803) (-14.8425, -4.9977) (-8.1192, -2.7212) knots -1 -1 -1 0 0 0
  line L106 (-8.1192, -2.7212) -> (-7.5025, -4.683)
  spline S105 degree 2 poles (-7.5025, -4.683) (-12.9817, -6.5867) (-13.65, -10.2696) knots -1 -1 -1 0 0 0
  line L107 (-13.65, -10.2696) -> (-13.7724, -10.6467)
  line L108 (-13.7724, -10.6467) -> (-11.3175, -10.6467)
  line L109 (-11.3175, -10.6467) -> (-11.3175, -10.0698)
  line L110 (-11.3175, -10.0698) -> (-9.2559, -10.0698)
  line L111 (-9.2559, -10.0698) -> (-9.2559, -17.1551)
  line L112 (-9.2559, -17.1551) -> (-20.89, -17.1551)
  line L113 (-20.89, -17.1551) -> (-20.89, -10.8154)
  spline S106 degree 2 poles (-20.89, -10.8154) (-20.89, -6.2032) (-23.4212, -3.7107) knots -1 -1 -1 0 0 0
  line L114 (-23.4212, -3.7107) -> (-21.9192, -2.3172)
  spline S107 degree 2 poles (-21.9192, -2.3172) (-18.8283, -5.7476) (-18.8283, -9.8721) knots -1 -1 -1 0 0 0
  line L115 (-18.8283, -9.8721) -> (-18.8283, -10.6467)
  line L116 (-18.8283, -10.6467) -> (-15.5741, -10.6467)
  line L117 (-15.5741, -10.6467) -> (-15.5333, -10.3803)
  line L118 (-133.4456, -25.6468) -> (-134.4941, -25.6468)
  line L119 (-134.4941, -25.6468) -> (-135.1301, -26.9876)
  spline S108 degree 2 poles (-135.1301, -26.9876) (-135.7232, -28.2338) (-136.342, -29.0503) knots -1 -1 -1 0 0 0
  spline S109 degree 2 poles (-136.342, -29.0503) (-136.8921, -29.7809) (-137.7516, -30.0216) knots -1 -1 -1 0 0 0
  spline S110 degree 2 poles (-137.7516, -30.0216) (-137.1241, -30.3739) (-136.8147, -30.8209) knots -1 -1 -1 0 0 0
  spline S111 degree 2 poles (-136.8147, -30.8209) (-136.5655, -31.1647) (-136.2905, -31.9382) knots -1 -1 -1 0 0 0
  spline S112 degree 2 poles (-136.2905, -31.9382) (-135.8521, -33.1673) (-135.6286, -33.5626) knots -1 -1 -1 0 0 0
  spline S113 degree 2 poles (-135.6286, -33.5626) (-135.1731, -34.3791) (-133.9011, -34.3447) knots -1 -1 -1 0 0 0
  line L120 (-133.9011, -34.3447) -> (-133.5401, -34.3362)
  line L121 (-133.5401, -34.3362) -> (-133.5401, -36.2184)
  spline S114 degree 2 poles (-133.5401, -36.2184) (-133.8237, -36.2098) (-133.9097, -36.2098) knots -1 -1 -1 0 0 0
  spline S115 degree 2 poles (-133.9097, -36.2098) (-135.8091, -36.2098) (-136.6085, -35.591) knots -1 -1 -1 0 0 0
  spline S116 degree 2 poles (-136.6085, -35.591) (-137.3304, -35.0323) (-138.0524, -33.1673) knots -1 -1 -1 0 0 0
  spline S117 degree 2 poles (-138.0524, -33.1673) (-138.6111, -31.7405) (-138.7228, -31.5514) knots -1 -1 -1 0 0 0
  spline S118 degree 2 poles (-138.7228, -31.5514) (-139.1783, -30.8638) (-140.1323, -30.7693) knots -1 -1 -1 0 0 0
  line L122 (-140.1323, -30.7693) -> (-140.1323, -36.1325)
  line L123 (-140.1323, -36.1325) -> (-142.6764, -36.1325)
  line L124 (-142.6764, -36.1325) -> (-142.6764, -23.5325)
  line L125 (-142.6764, -23.5325) -> (-140.1323, -23.5325)
  line L126 (-140.1323, -23.5325) -> (-140.1323, -29.0503)
  spline S119 degree 2 poles (-140.1323, -29.0503) (-139.4018, -29.0417) (-139.0236, -28.6808) knots -1 -1 -1 0 0 0
  spline S120 degree 2 poles (-139.0236, -28.6808) (-138.8001, -28.4573) (-138.3704, -27.6494) knots -1 -1 -1 0 0 0
  spline S121 degree 2 poles (-138.3704, -27.6494) (-138.1126, -27.1595) (-138.0524, -27.0563) knots -1 -1 -1 0 0 0
  spline S122 degree 2 poles (-138.0524, -27.0563) (-137.9407, -26.8587) (-137.9063, -26.7899) knots -1 -1 -1 0 0 0
  line L127 (-137.9063, -26.7899) -> (-136.4022, -23.5325)
  line L128 (-136.4022, -23.5325) -> (-135.5599, -23.5325)
  line L129 (-135.5599, -23.5325) -> (-135.5599, -20.7821)
  line L130 (-135.5599, -20.7821) -> (-133.4456, -20.7821)
  line L131 (-133.4456, -20.7821) -> (-133.4456, -25.6468)
  line L132 (-148, -42) -> (0, -42)
  line L133 (0, -42) -> (0, 0)
  line L134 (0, 0) -> (-148, 0)
  line L135 (-148, 0) -> (-148, -42)
  line L136 (-140, -5) -> (-8, -5)
  line L137 (-8, -5) -> (-8, -37)
  line L138 (-8, -37) -> (-140, -37)
  line L139 (-140, -37) -> (-140, -5)
  dimension "d10" = 8
  dimension "d11" = 5
  dimension "d12" = 5
  dimension "d13" = 8
  constraint horizontal L136
  constraint vertical L137
  constraint horizontal L138
  constraint vertical L139
  measures "d10" distance of L133 L137
  measures "d11" distance of L134 L136
  measures "d12" distance of L132 L138
  measures "d13" distance of L135 L139
extrude "Extrude2" add sketch "Sketch1" against normal up to surface (10 mm away) separate body contours L4 L5 L6 L7 S0 S1 S2 S3 L8 L9 L10 L11 L12 S4 S5 S6 S7 S8 L13 L14 S9 S10 S11 S12 S13 S14 L15 L16 L17 | L18 L19 L20 S15 S16 S17 S18 S19 L21 L22 L23 S20 S21 S22 S23 | L26 L27 L28 L29 L30 L31 S32 S33 S34 S35 L32 L33 S36 S37 L34 L35 | L36 L37 L38 L39 L40 L41 L42 L43 | L44 L45 L46 L47 L48 L49 L50 | S38 S39 S40 S41 S42 S43 S44 S45 S46 L51 S47 S48 S49 S50 S51 L52 L53 L54 S52 S53 S54 S55 S56 S57 L55 | L56 L57 L58 L59 L60 L61 S58 S59 S60 S61 L62 L63 S62 S63 L64 L65 | L66 L67 L68 L69 L70 L71 L72 L73 | L74 L75 L76 L77 L78 L79 L80 | L81 L82 L83 L84 S64 S65 S66 S67 L85 L86 L87 L88 L89 S68 S69 S70 S71 S72 L90 L91 S73 S74 S75 S76 S77 S78 L92 L93 L94 | S79 S80 S81 S82 S83 S84 S85 S86 S87 L95 S88 S89 S90 S91 S92 L96 L97 L98 S93 S94 S95 S96 S97 S98 L99 | L100 L101 L102 L103 L104 L105 L106 L107 L108 L109 L110 L111 L112 L113 | L114 S99 S100 S101 S102 S103 S104 S105 S106 L115 L116 L117 L118 L119 L120 | S114 S115 S116 S117 S118 S119 S120 S121 S122 L128 S123 S124 S125 S126 S127 L129 L130 L131 S128 S129 S130 S131 S132 S133 L132 | L133 L134 S134 L135 S135 L136 L137 L138 L139 L140 L141 L142 S136 L143 S137 L144 makes body 6 at (-45.7756, 13.9235, 0) makes body 7 at (-69.5345, 37.7512, -3.3333) makes body 8 at (-103.6645, 37.7512, -3.3333) makes body 9 at (-142.6764, 27.7325, -6.6667) makes body 10 at (-103.0973, 27.022, -3.3333) makes body 11 at (-68.9673, 27.022, -3.3333) makes body 12 at (-51.3221, 3.8675, -3.3333) makes body 13 at (-30.6649, 10.2626, 0) makes body 14 at (-79.1005, 8.0675, -6.6667) makes body 15 at (-91.9373, 29.9275, 0) makes body 16 at (-127.0911, 28.5862, 0) makes body 17 at (-108.555, 31.9325, -6.6667) makes body 18 at (-74.425, 31.9325, -6.6667) makes body 19 at (-65.1559, 10.2626, 0) makes body 20 at (-17.012, 17.1551, -3.3333)
extrude "Extrude3" add sketch "Sketch2" along normal blind 65 contours L17 L18 L19 L20 L21 L22 L138 | L37 L38 L39 L40 L41 L42 L138 | S118 L122 L123 L124 L125 L126 S119 L139 | L49 L50 L51 L136 | S104 L106 S105 L136 | L52 L53 L54 L55 L56 L136 | S106 L114 S107 L136 | S72 S73 S74 S75 L136 | S100 S101 S102 S103 L136 | L94 L95 L96 L136 | L83 L84 S76 S77 L136 | L132 L133 L134 L135 bodies 4 6 7 8 9 12 13 14 19 20
equation "d12 = d11"
equation "d13 = d10"
